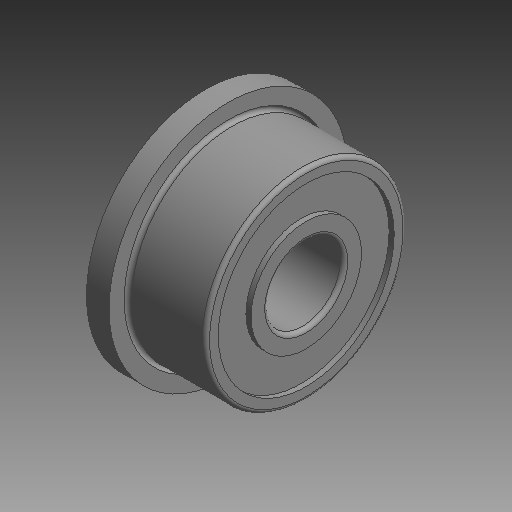
# Autodesk Inventor part: FL693ZZ
Saved by Autodesk Inventor 2019 (Build 230136000, 136)
## iProperties
Category: PARTsolutions
Company: MISUMI
Part Number: FL693ZZ
Material: 일반
Catalog Web Link: www.cadenas.de
Description: FL6 _ _ ZZ, FL6 _ _ AZZ, SFL6 _ _ ZZ, SFL6 _ _ AZZ, MFL1 _ _ ZZ, SMFL1 _ _ ZZ-Flanged Ball Bearings (Small Diameter, Deep Groove) - Double Shield Type
Vendor: MISUMI
Document SubType Name: Modeling
Designer: partserver
Manufacturer: MISUMI
Mass: 0.180492 g
Surface Area: 2.91616 cm^2
Volume: 0.180492 cm^3
Density: 1 g/cm^3
Appearance: PSOLRGB-175-175-175
PSOL_IDENT_0: {$CADENAS_DATA\23d-libs\misumi\metric\12_bearing_holders\sfl608zz.prj},228 {VTYP=3D},{NB=FL693ZZ},{L
PSOL_IDENT_1: INA=FL693ZZ},{NN=FL6 _ _ ZZ, FL6 _ _ AZZ, SFL6 _ _ ZZ, SFL6 _ _ AZZ, MFL1 _ _ ZZ, SMFL1 _ _ ZZ},{DAT
PSOL_IDENT_2: E=09.09.2019 15:26:56},{GEOMDATE=16.08.2017 04:27:24},{VERSION=},{LINEID=20},{WBVAR=MAT},{WBNUMERIC=
PSOL_IDENT_3: }  {NB=FL693ZZ},{LINA=FL693ZZ},{KT=DUMMY},{PN=FL693ZZ},{MAT=},{MAT1= '', '52100 Bearing Steel', 'S',
PSOL_IDENT_4: '440C Stainless Steel'},{BN=693ZZ},{DD=3.0},{AA=3.6000},{BB=0.5000},{C1=0.7000},{D=8},{B=4.0},{D1=9
PSOL_IDENT_5: .5},{C=0.9},{RR=0.15},{CR=560},{COR=180},{CRS=560},{CRSS=474},{CORS=180},{CORSS=144},{DS=4.20},{R=0.
PSOL_IDENT_6: 15},{MASS=0.72},{MAT11=1},{MMMM=}
NB: FL693ZZ
NN: FL6 _ _ ZZ, FL6 _ _ AZZ, SFL6 _ _ ZZ, SFL6 _ _ AZZ, MFL1 _ _ ZZ, SMFL1 _ _ ZZ
NT: Flanged Ball Bearings (Small Diameter, Deep Groove) - Double Shield Type
NBSYN: $PN.
LINA: FL693ZZ
CATALOG: Misumi
PN: FL693ZZ
MAT: 52100 Bearing Steel
BN: 693ZZ
DD: 3
D: 8
B: 4
D1: 9.5
C: 0.9
RR: 0.15
CR: 560
COR: 180
DS: 4.2
R: 0.15
MASS: 0.72
SUPPLIER: MISUMI
ARTICLENO: FL693ZZ
BOMINFO: FL693ZZ
CREATOR: CADENAS GmbH
Title: FL693ZZ
Author: Cadenas PARTsolutions
Comments: Flanged Ball Bearings (Small Diameter, Deep Groove) - Double Shield Type
Autodesk Inventor part; units mm, degrees
sketch "Sketch_1" plane through (0, 0, 0) normal (0, 0, 1) x (1, 0, 0)
  line L0 (8, 0) -> (-8, 0)
  arc A0 (0, 1.65) -> (0.15, 1.5) centre (0.15, 1.65) ccw
  line L1 (0.15, 1.5) -> (3.85, 1.5)
  arc A1 (3.85, 1.5) -> (4, 1.65) centre (3.85, 1.65) ccw
  line L2 (4, 1.65) -> (4, 2.2)
  line L3 (4, 2.2) -> (3.8, 2.2)
  line L4 (3.8, 2.2) -> (3.8, 3.5)
  line L5 (3.8, 3.5) -> (4, 3.5)
  line L6 (4, 3.5) -> (4, 4.75)
  line L7 (4, 4.75) -> (3.1, 4.75)
  line L8 (3.1, 4.75) -> (3.1, 4.15)
  arc A2 (2.95, 4) -> (3.1, 4.15) centre (3.1, 4) ccw
  line L9 (2.95, 4) -> (0.15, 4)
  arc A3 (0.15, 4) -> (0, 3.85) centre (0.15, 3.85) ccw
  line L10 (0, 3.85) -> (0, 3.5)
  line L11 (0, 3.5) -> (0.2, 3.5)
  line L12 (0.2, 3.5) -> (0.2, 2.2)
  line L13 (0.2, 2.2) -> (0, 2.2)
  line L14 (0, 2.2) -> (0, 1.65)
  constraints: 30 end point, 8 point on circle, 4 centre point
revolve "Revolution1" add sketch "Sketch_1" angle 360 about axis through (8, 0, 0) along (1, 0, 0)
ref_plane "to_housing_XY" through (0, 0, 0) normal (1, 0, 0) x (0, 0, -1)
ref_plane "to_housing_YZ" through (0, 0, 0) normal (0, 0, -1) x (0, 1, 0)
ref_plane "to_housing_ZX" through (0, 0, 0) normal (0, 1, 0) x (1, 0, 0)
body "Solid1"
